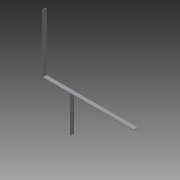
# Autodesk Inventor part: ArmTest
Saved by Autodesk Inventor 2013 (Build 170138000, 138)
## iProperties
Created: 2014-01-09
Part Number: ArmTest
Material: Generic
Document SubType Name: Modeling
Designer: 215152
Density: 1 g/cm^3
Author: 215152
Autodesk Inventor part; units mm, degrees
ref_plane "YZ Plane" through (0, 0, 0) normal (1, 0, 0) x (0, 1, 0)
ref_plane "XZ Plane" through (0, 0, 0) normal (0, 1, 0) x (-1, 0, 0)
ref_plane "XY Plane" through (0, 0, 0) normal (0, 0, 1) x (1, 0, 0)
sketch "Sketch1" plane through (0, 0, 0) normal (0, 0, 1) x (1, 0, 0)
  line L0 (0, 0) -> (127, 0)
  line L1 (127, 0) -> (127, 76.2)
  line L2 (127, 76.2) -> (0, 76.2)
  line L3 (0, 76.2) -> (0, 0)
  line L4 (0, 0) -> (-50.8, 0)
  line L5 (-50.8, 0) -> (-50.8, 76.2)
  line L6 (-50.8, 76.2) -> (0, 76.2)
  line L7 (0, 76.2) -> (0, 0)
  line L8 (-50.8, 76.2) -> (127, 76.2)
  line L9 (127, 76.2) -> (127, 88.9)
  line L10 (127, 88.9) -> (-50.8, 88.9)
  line L11 (-50.8, 88.9) -> (-50.8, 76.2)
  line L12 (-50.8, 88.9) -> (-47.625, 88.9)
  line L13 (-47.625, 88.9) -> (-47.625, 495.3)
  line L14 (-47.625, 495.3) -> (-50.8, 495.3)
  line L15 (-50.8, 495.3) -> (-50.8, 88.9)
  line L16 (-50.8, 88.9) -> (584.2, 88.9)
  line L17 (584.2, 88.9) -> (584.2, 92.075)
  line L18 (584.2, 92.075) -> (-50.8, 92.075)
  line L19 (-50.8, 92.075) -> (-50.8, 88.9)
  line L20 (127, 76.2) -> (139.7, 76.2)
  line L21 (139.7, 76.2) -> (139.7, 88.9)
  line L22 (139.7, 88.9) -> (127, 88.9)
  line L23 (127, 88.9) -> (127, 76.2)
  line L24 (139.7, 88.9) -> (142.875, 88.9)
  line L25 (142.875, 88.9) -> (142.875, -165.1)
  line L26 (142.875, -165.1) -> (139.7, -165.1)
  line L27 (139.7, -165.1) -> (139.7, 88.9)
  dimension "d11" = 127
  dimension "d12" = 76.2
  dimension "d13" = 50.8
  dimension "d14" = 76.2
  dimension "d15" = 177.8
  dimension "d16" = 12.7
  dimension "d17" = 3.175
  dimension "d18" = 406.4
  dimension "d19" = 635
  dimension "d20" = 3.175
  dimension "d21" = 12.7
  dimension "d22" = 12.7
  dimension "d23" = 3.175
  dimension "d24" = 254
  constraints: 56 end point, 14 parallel, 7 horizontal, 7 perpendicular
  measures "d11" distance of L2.end L1.end
  measures "d12" distance of L1.end L0.end
  measures "d13" distance of L5.end L6.end
  measures "d14" distance of L4.end L5.end
  measures "d15" distance of L10.end L9.end
  measures "d16" distance of L9.end L8.end
  measures "d17" distance of L14.end L13.end
  measures "d18" distance of L13.end L12.end
  measures "d19" distance of L18.end L17.end
  measures "d20" distance of L17.end L16.end
  measures "d21" distance of L22.end L21.end
  measures "d22" distance of L21.end L20.end
  measures "d23" distance of L25.end L26.end
  measures "d24" distance of L24.end L25.end
extrude "Extrusion1" add sketch "Sketch1" against normal blind 101.6 contours L10 L13 L18 L17 L16 | L21 L16 L25 L26 L27 | L15 L18 L13 L10 | L15 L14 L13 L18
sketch "Sketch2" plane through (0, 0, 0) normal (0, 0, 1) x (1, 0, 0)
  line L0 (-50.8, 88.9) -> (139.7, 88.9) projected
  line L1 (139.7, 88.9) -> (139.7, -165.1) projected
  line L2 (139.7, -165.1) -> (142.875, -165.1) projected
  line L3 (142.875, -165.1) -> (142.875, 88.9) projected
  line L4 (142.875, 88.9) -> (584.2, 88.9) projected
  line L5 (584.2, 88.9) -> (584.2, 92.075) projected
  line L6 (584.2, 92.075) -> (-47.625, 92.075) projected
  line L7 (-47.625, 92.075) -> (-47.625, 495.3) projected
  line L8 (-47.625, 495.3) -> (-50.8, 495.3) projected
  line L9 (-50.8, 495.3) -> (-50.8, 88.9) projected
  point P0 (0, 0)
extrude "Extrusion2" cut sketch "Sketch2" against normal blind 76.2
body "Solid1"
